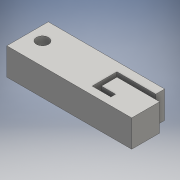
# Autodesk Inventor part: opto mount
Saved by Autodesk Inventor 2016 SP1 (Build 200210100, 210)
## iProperties
Created: 2017-05-11
Part Number: opto mount
Material: Generic
Document SubType Name: Modeling
Designer: Cole
Density: 1 g/cm^3
Appearance: Default
Author: Cole
Autodesk Inventor part; units mm, degrees
ref_plane "YZ Plane" through (0, 0, 0) normal (1, 0, 0) x (0, 1, 0)
ref_plane "XZ Plane" through (0, 0, 0) normal (0, 1, 0) x (-1, 0, 0)
ref_plane "XY Plane" through (0, 0, 0) normal (0, 0, 1) x (1, 0, 0)
sketch "Sketch1" plane through (0, 0, 0) normal (0, 0, 1) x (1, 0, 0)
  line L0 (-20, -0.7) -> (-20, 10)
  line L1 (0, 7.7) -> (0, 1.3)
  circle A0 centre (-16.5, 5) radius 1.5606
  line L2 (1.2, 6.5) -> (12.2, 6.5)
  line L3 (1.2, 2.5) -> (4.8537, 2.5)
  line L4 (1.2, 6.5) -> (1.2, 2.5)
  line L5 (0, 1.3) -> (4.8537, 1.3)
  line L6 (4.8537, 2.5) -> (4.8537, 1.3)
  line L7 (12.2, -0.7) -> (12.2, 6.5)
  line L8 (0, 7.7) -> (10, 7.7)
  line L9 (10, 7.7) -> (10, 10)
  line L10 (-20, -0.7) -> (12.2, -0.7)
  line L11 (-20, 10) -> (10, 10)
  dimension "d0" = 16.5
  dimension "d7" = 1.2
  dimension "d9" = 1.2
  dimension "d10" = 11
  dimension "d12" = 1.2
  dimension "d13" = 4
  dimension "d14" = 2
  dimension "d17" = 5
  constraints: 24 end point, 1 centre point, 1 horizontal, 1 parallel, 1 perpendicular, 1 vertical
  measures "d0" distance from line of L1 A0.centre
  measures "d7" distance between parallel lines of L1 L4
  measures "d9" distance between parallel lines of L5 L3
  measures "d10" distance between parallel lines of L7 L4
  measures "d12" distance between parallel lines of L2 L8
  measures "d13" distance between parallel lines of L3 L2
  measures "d14" distance between parallel lines of L10 L5
  measures "d17" distance from line of L11 A0.centre
extrude "Extrusion1" add sketch "Sketch1" along normal blind 7
sketch "Sketch2" plane through (0, 0, 0) normal (0, 0, -1) x (-1, 0, 0)
  line L0 (20, 10) -> (2.1389, 10)
  line L1 (2.1389, 10) -> (2.1389, 9)
  line L2 (2.1389, 9) -> (20, 9)
  line L3 (20, 9) -> (20, 10)
  line L4 (20, 10) -> (-10, 10) projected
  line L5 (20, -0.7) -> (20, 10) projected
  point P0 (0, 0)
  dimension "d18" = 1
  constraints: 8 end point, 2 collinear, 2 parallel, 1 horizontal, 1 perpendicular
  measures "d18" distance between parallel lines of L2 L0
extrude "Extrusion2" add sketch "Sketch2" along normal blind 2
body "Solid1"
